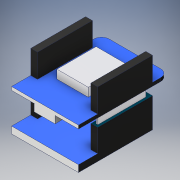
# Autodesk Inventor part: Wemos
Saved by Autodesk Inventor 2019 (Build 230136000, 136)
## iProperties
Created: 2019-02-11
Part Number: Wemos
Material: Generic
Document SubType Name: Modeling
Designer: izsoandras
Density: 1 g/cm^3
Appearance: PTFE
Author: izsoandras
Autodesk Inventor part; units mm, degrees
ref_plane "YZ Plane" through (0, 0, 0) normal (1, 0, 0) x (0, 1, 0)
ref_plane "XZ Plane" through (0, 0, 0) normal (0, 1, 0) x (-1, 0, 0)
ref_plane "XY Plane" through (0, 0, 0) normal (0, 0, 1) x (1, 0, 0)
sketch "Sketch1" plane through (0, 0, 0) normal (0, 1, 0) x (-1, 0, 0)
  line L0 (2.4457, 9.8333) -> (-23.1743, 9.8333)
  line L1 (-23.1743, 9.8333) -> (-23.1743, -18.5067)
  line L2 (-23.1743, -18.5067) -> (2.4457, -18.5067)
  line L3 (2.4457, -18.5067) -> (2.4457, 9.8333)
  point P0 (0, 0)
  dimension "d0" = 28.34
  dimension "d1" = 25.62
  constraints: 8 end point, 2 parallel, 1 horizontal, 1 perpendicular
  measures "d0" distance of L2.end L0.start
  measures "d1" distance of L0.start L0.end
extrude "Extrusion1" add sketch "Sketch1" along normal blind 2.6
sketch "Sketch2" plane through (0, 2.6, 0) normal (0, 1, 0) x (1, 0, 0)
  line L0 (23.1743, 18.5067) -> (-2.4457, 18.5067) projected
  line L1 (-2.4457, 18.5067) -> (0.1443, 18.5067)
  line L2 (0.1443, 18.5067) -> (0.1443, -2.4933)
  line L3 (0.1443, -2.4933) -> (-2.4457, -2.4933)
  line L4 (-2.4457, -2.4933) -> (-2.4457, 18.5067)
  point P0 (0, 0)
  dimension "d4" = 21
  dimension "d5" = 2.59
  constraints: 8 end point, 2 parallel, 1 horizontal, 1 perpendicular
  measures "d4" distance of L1.end L2.end
  measures "d5" distance of L2.end L3.end
extrude "Extrusion2" add sketch "Sketch2" along normal blind 8.7
sketch "Sketch3" plane through (0, 2.6, 0) normal (0, 1, 0) x (1, 0, 0)
  line L0 (23.1743, 18.5067) -> (20.5843, 18.5067)
  line L1 (20.5843, 18.5067) -> (20.5843, -2.4933)
  line L2 (20.5843, -2.4933) -> (23.1743, -2.4933)
  line L3 (23.1743, -2.4933) -> (23.1743, 18.5067)
  point P0 (0, 0)
  dimension "d8" = 21
  dimension "d9" = 2.59
  constraints: 8 end point, 2 parallel, 1 horizontal, 1 perpendicular
  measures "d8" distance of L0.end L1.end
  measures "d9" distance of L1.end L2.end
extrude "Extrusion3" add sketch "Sketch3" along normal blind 8.7
sketch "Sketch4" plane through (0, 11.3, 0) normal (0, 1, 0) x (1, 0, 0)
  line L0 (-1.4241, 16.7919) -> (-0.8041, 16.7919)
  line L1 (-0.8041, 16.7919) -> (-0.8041, -1.6081)
  line L2 (-0.8041, -1.6081) -> (-1.4241, -1.6081)
  line L3 (-1.4241, -1.6081) -> (-1.4241, 16.7919)
  line L4 (21.7236, 16.7919) -> (22.3436, 16.7919)
  line L5 (22.3436, 16.7919) -> (22.3436, -1.6081)
  line L6 (22.3436, -1.6081) -> (21.7236, -1.6081)
  line L7 (21.7236, -1.6081) -> (21.7236, 16.7919)
  point P0 (0, 0)
  dimension "d14" = 18.4
  dimension "d15" = 0.62
  dimension "d16" = 18.4
  dimension "d17" = 0.62
  constraints: 16 end point, 4 parallel, 2 horizontal, 2 perpendicular
  measures "d14" distance of L0.end L1.end
  measures "d15" distance of L0.start L0.end
  measures "d16" distance of L6.end L4.start
  measures "d17" distance of L4.start L4.end
extrude "Extrusion4" add sketch "Sketch4" along normal blind 3.12
sketch "Sketch5" plane through (0, 14.42, 0) normal (0, 1, 0) x (1, 0, 0)
  line L0 (-2.4457, -9.8333) -> (23.1743, -9.8333) projected
  line L1 (23.1743, -9.8333) -> (23.1743, -2.4933) projected
  line L2 (-2.4457, -9.8333) -> (23.1743, -9.8333)
  line L3 (23.1743, -9.8333) -> (23.1743, 21.5867)
  line L4 (20.1743, 24.5867) -> (0.5543, 24.5867)
  line L5 (-2.4457, 21.5867) -> (-2.4457, -9.8333)
  arc A0 (0.5543, 24.5867) -> (-2.4457, 21.5867) centre (0.5543, 21.5867) ccw
  arc A1 (23.1743, 21.5867) -> (20.1743, 24.5867) centre (20.1743, 21.5867) ccw
  point P0 (0, 0)
  point P1 (-2.4457, 24.5867)
  dimension "d18" = 34.42
  dimension "d19" = 3
  constraints: 8 end point, 4 point on circle, 4 tangent, 2 centre point, 2 parallel, 2 point on line, 1 equal radius, 1 horizontal, 1 perpendicular
  measures "d18" distance of point (-2.446, 24.587) L0.start
  measures "d19" radius of A0
extrude "Extrusion5" add sketch "Sketch5" along normal blind 1.3
sketch "Sketch6" plane through (0, 15.72, 0) normal (0, 1, 0) x (1, 0, 0)
  line L0 (-2.4457, -2.4933) -> (0.1443, -2.4933) projected
  line L1 (0.1443, 18.5067) -> (-2.4457, 18.5067) projected
  line L2 (-2.4457, -2.4933) -> (0.1443, -2.4933)
  line L3 (0.1443, -2.4933) -> (0.1443, 18.5067)
  line L4 (0.1443, 18.5067) -> (-2.4457, 18.5067)
  line L5 (-2.4457, 18.5067) -> (-2.4457, -2.4933)
  line L6 (23.1743, -2.4933) -> (20.5843, -2.4933) projected
  line L7 (20.5843, 18.5067) -> (0.1443, 18.5067) projected
  line L8 (23.1743, -2.4933) -> (20.5843, -2.4933)
  line L9 (20.5843, -2.4933) -> (20.5843, 18.5067)
  line L10 (20.5843, 18.5067) -> (23.1743, 18.5067)
  line L11 (23.1743, 18.5067) -> (23.1743, -2.4933)
  point P0 (0, 0)
  constraints: 16 end point, 4 parallel, 2 horizontal, 2 perpendicular
extrude "Extrusion6" add sketch "Sketch6" along normal blind 9
sketch "Sketch7" plane through (0, 15.72, 0) normal (0, 1, 0) x (1, 0, 0)
  line L0 (3.7943, 16.2867) -> (15.7943, 16.2867)
  line L1 (15.7943, 16.2867) -> (15.7943, 1.2867)
  line L2 (15.7943, 1.2867) -> (3.7943, 1.2867)
  line L3 (3.7943, 1.2867) -> (3.7943, 16.2867)
  line L4 (20.5843, 18.5067) -> (20.5843, -2.4933) projected
  line L5 (-2.4457, -9.8333) -> (23.1743, -9.8333) projected
  point P0 (0, 0)
  dimension "d24" = 15
  dimension "d25" = 12
  dimension "d28" = 4.79
  dimension "d29" = 11.12
  constraints: 8 end point, 2 parallel, 1 horizontal, 1 perpendicular
  measures "d24" distance of L2.end L0.start
  measures "d25" distance of L1.end L2.end
  measures "d28" distance between parallel lines of L4 L1
  measures "d29" distance between parallel lines of L5 L2
extrude "Extrusion7" add sketch "Sketch7" along normal blind 3.3
sketch "Sketch8" plane through (0, 14.42, 0) normal (0, -1, 0) x (1, 0, 0)
  line L0 (-2.4457, 9.8333) -> (23.1743, 9.8333) projected
  line L1 (14.1743, 9.8333) -> (6.2543, 9.8333)
  line L2 (6.2543, 9.8333) -> (6.2543, 4.2333)
  line L3 (6.2543, 4.2333) -> (14.1743, 4.2333)
  line L4 (14.1743, 4.2333) -> (14.1743, 9.8333)
  line L5 (23.1743, 9.8333) -> (23.1743, -21.5867) projected
  point P0 (0, 0)
  dimension "d30" = 9
  dimension "d31" = 7.92
  dimension "d32" = 5.6
  constraints: 8 end point, 2 parallel, 1 horizontal, 1 perpendicular, 1 point on line
  measures "d30" distance between parallel lines of L5 L4
  measures "d31" distance of L2.end L3.end
  measures "d32" distance of L1.end L2.end
extrude "Extrusion8" add sketch "Sketch8" along normal blind 2.78
equation "\"d16\" = d14"
equation "\"d17\" = d15"
body "Solid1"
